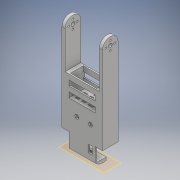
# Autodesk Inventor part: arm_1
Saved by Autodesk Inventor 2018 (Build 220112000, 112)
## iProperties
Created: 2018-02-05
Part Number: arm_1
Material: Genérico
Document SubType Name: Modeling
Designer: se_ma
Density: 1 g/cm^3
Appearance: Valor por defecto
Author: se_ma
Autodesk Inventor part; units mm, degrees
ref_plane "YZ Plane" through (0, 0, 0) normal (1, 0, 0) x (0, 1, 0)
ref_plane "XZ Plane" through (0, 0, 0) normal (0, 1, 0) x (-1, 0, 0)
ref_plane "XY Plane" through (0, 0, 0) normal (0, 0, 1) x (1, 0, 0)
sketch "Boceto1" plane through (0, 0, 0) normal (0, 1, 0) x (-1, 0, 0)
  line L0 (0, 0) -> (60, 0)
  line L1 (60, 0) -> (60, -80)
  line L2 (60, -80) -> (0, -80)
  line L3 (0, -80) -> (0, 0)
  dimension "d0" = 60
  dimension "d1" = 80
  constraints: 8 end point, 2 parallel, 1 horizontal, 1 perpendicular
  measures "d0" distance of L1.end L2.end
  measures "d1" distance of L0.end L1.end
extrude "Extrusión1" add sketch "Boceto1" along normal blind 25
sketch "Boceto2" plane through (-60, 0, 0) normal (0, 0, 1) x (1, 0, 0)
  line L0 (0, 25) -> (60, 25) projected
  line L1 (30, 25) -> (30, 23)
  line L2 (60, 0) -> (0, 0) projected
  line L3 (30, 0) -> (30, 2)
  line L4 (0, 0) -> (0, 25) projected
  line L5 (60, 0) -> (60, 25) projected
  line L6 (30, 23) -> (9, 23)
  line L7 (9, 2) -> (30, 2)
  line L8 (30, 23) -> (51, 23)
  line L9 (51, 2) -> (30, 2)
  line L10 (9, 23) -> (9, 19.5)
  line L11 (9, 2) -> (9, 5.5)
  arc A0 (9, 19.5) -> (1, 12.5) centre (7.9996, 12.5719) ccw
  arc A1 (1, 12.5) -> (9, 5.5) centre (7.9996, 12.4281) ccw
  line L12 (51, 23) -> (51, 19.5)
  line L13 (51, 2) -> (51, 5.5)
  arc A2 (59, 12.5) -> (51, 19.5) centre (52.0004, 12.5719) ccw
  arc A3 (51, 5.5) -> (59, 12.5) centre (52.0004, 12.4281) ccw
  dimension "d4" = 2
  dimension "d5" = 2
  dimension "d7" = 21
  dimension "d12" = 3.5
  dimension "d13" = 3.5
  dimension "d15" = 7
  dimension "d16" = 7
  dimension "d17" = 3.5
  dimension "d18" = 3.5
  dimension "d19" = 7
  dimension "d20" = 7
  constraints: 20 end point, 8 point on circle, 5 vertical, 4 centre point, 2 midpoint, 2 point on line, 1 horizontal
  measures "d4" distance of L1.start L1.end
  measures "d5" distance of L3.start L3.end
  measures "d7" distance of L1.end L8.end
  measures "d12" distance of L6.end L10.end
  measures "d13" distance of L7.start L11.end
  measures "d15" radius of A0
  measures "d16" radius of A1
  measures "d17" distance of L8.end L12.end
  measures "d18" distance of L9.start L13.end
  measures "d19" radius of A2
  measures "d20" radius of A3
extrude "Extrusión2" cut sketch "Boceto2" against normal blind 80 contours L8 L12 A2 A3 L13 L9 L7 L11 A1 A0 L10 L6
move faces "Desplazar1" translate (-1, 0, 0) faces at (-60, 8.3333, -26.6667)
move faces "Desplazar2" translate (1, 0, 0) faces at (0, 8.3333, -53.3333)
sketch "Boceto3" plane through (1, 0, 0) normal (1, 0, 0) x (0, 0, -1)
  line L0 (0, 0) -> (80, 0) projected
  line L1 (80, 0) -> (80, 25) projected
  line L2 (80, 0) -> (80, 25)
  line L3 (80, 25) -> (-60, 25)
  circle A0 centre (-60, 19.5) radius 1.5
  circle A1 centre (-67, 12.5) radius 1.5
  circle A2 centre (-60, 5.5) radius 1.5
  circle A3 centre (-53, 12.5) radius 1.5
  circle A4 centre (-60, 12.5) radius 3
  line L4 (80, 0) -> (-60, 0)
  arc A5 (-60, 25) -> (-60, 0) centre (-60, 12.5) ccw
  dimension "d29" = 25
  dimension "d30" = 140
  dimension "d35" = 3
  dimension "d36" = 3
  dimension "d37" = 3
  dimension "d38" = 3
  dimension "d39" = 6
  constraints: 6 centre point, 6 end point, 2 point on circle, 1 coincident, 1 horizontal, 1 perpendicular, 1 vertical
  measures "d29" distance of L0.end L1.end
  measures "d30" distance of L1.end L3.end
  measures "d35" diameter of A0
  measures "d36" diameter of A1
  measures "d37" diameter of A2
  measures "d38" diameter of A3
  measures "d39" diameter of A4
extrude "Extrusión3" add sketch "Boceto3" along normal blind 5
sketch "Boceto5" plane through (-61, 0, -80) normal (-1, 0, 0) x (0, 0, 1)
  line L0 (0, 0) -> (0, 25) projected
  line L1 (0, 0) -> (0, 25)
  line L2 (0, 25) -> (140, 25)
  line L3 (0, 0) -> (140, 0)
  circle A0 centre (140, 12.5) radius 3 projected
  circle A1 centre (140, 12.5) radius 3
  circle A2 centre (140, 19.5) radius 1.5
  circle A3 centre (133, 12.5) radius 1.5
  circle A4 centre (147, 12.5) radius 1.5
  circle A5 centre (140, 5.5) radius 1.5
  arc A6 (140, 0) -> (140, 25) centre (140, 12.5) ccw
  point P0 (80, 0)
  dimension "d52" = 3
  dimension "d53" = 3
  dimension "d54" = 3
  dimension "d55" = 3
  constraints: 6 centre point, 6 end point, 2 coincident, 2 point on circle, 1 horizontal, 1 perpendicular, 1 vertical
  measures "d52" diameter of A2
  measures "d53" diameter of A3
  measures "d54" diameter of A4
  measures "d55" diameter of A5
extrude "Extrusión4" add sketch "Boceto5" along normal blind 5
sketch "Boceto7" plane through (6, 0, -80) normal (0, 0, -1) x (-1, 0, 0)
  line L0 (57, 2) -> (15, 2) projected
  line L1 (57, 2) -> (65, 2)
  line L2 (65, 2) -> (65, 23)
  line L3 (57, 23) -> (15, 23) projected
  line L4 (65, 23) -> (57, 23)
  line L5 (57, 23) -> (57, 2)
  line L6 (15, 2) -> (7, 2)
  line L7 (7, 2) -> (7, 23)
  line L8 (7, 23) -> (15, 23)
  line L9 (15, 2) -> (15, 5.5) projected
  line L10 (15, 2) -> (15, 23)
  point P0 (6, 0)
  dimension "d60" = 8
  dimension "d61" = 21
  dimension "d62" = 8
  constraints: 16 end point, 5 perpendicular, 2 horizontal
  measures "d60" distance of L0.start L1.end
  measures "d61" distance of L1.end L2.end
  measures "d62" distance of L0.end L6.end
extrude "Extrusión5" add sketch "Boceto7" against normal blind 80 contours L5 L4 L2 L1 | L6 L7 L8 L10 L9
move faces "Desplazar3" translate (3.5, 0, 0) faces at (-61, 12.5, 17.1667) (-66, 12.5, -36.1667)
move faces "Desplazar4" translate (-3.5, 0, 0) faces at (1, 12.5, 17.1667) (6, 12.5, -36.1667)
sketch "Boceto11" plane through (0, 25, 0) normal (0, 1, 0) x (1, 0, 0)
  line L0 (-62.5, 80) -> (2.5, 80) projected
  line L1 (-51, 0) -> (-51, 80) projected
  line L2 (-62.5, 80) -> (-51, 80)
  line L3 (-51, 80) -> (-51, 63)
  line L4 (-51, 0) -> (-51, 80) projected
  line L5 (-51, 63) -> (-9, 63)
  line L6 (-9, 0) -> (-9, 80) projected
  point P0 (0, 0)
  dimension "d104" = 17
  constraints: 6 end point, 2 perpendicular, 2 point on line
  measures "d104" distance of L1.end L3.end
extrude "Extrusión9" cut sketch "Boceto11" against normal blind 23
sketch "Boceto12" plane through (0, 25, 0) normal (0, 1, 0) x (1, 0, 0)
  line L0 (-51, 0) -> (-51, 63) projected
  line L1 (-51, 63) -> (-51, 0)
  line L2 (-9, 0) -> (-9, 63) projected
  line L3 (-51, 63) -> (-9, 63)
  line L4 (-9, 63) -> (-9, 0)
  line L5 (-9, 0) -> (-51, 0)
  point P0 (0, 0)
  constraints: 8 end point, 2 collinear, 1 horizontal, 1 perpendicular
extrude "Extrusión10" add sketch "Boceto12" against normal blind 23
sketch "Boceto13" plane through (0, 0, 0) normal (0, -1, 0) x (1, 0, 0)
  line L0 (-62.5, -80) -> (2.5, -80) projected
  line L1 (-51, -63) -> (-51, -80) projected
  line L2 (-62.5, -80) -> (-51, -80)
  line L3 (-51, -80) -> (-51, -103)
  line L4 (-51, -103) -> (-9, -103)
  line L5 (-9, -63) -> (-9, -80) projected
  line L6 (-9, -103) -> (-9, -80)
  line L7 (-9, -80) -> (-51, -80)
  point P0 (0, 0)
  dimension "d109" = 23
  dimension "d110" = 42
  constraints: 10 end point, 1 horizontal, 1 perpendicular, 1 vertical
  measures "d109" distance of L1.end L3.end
  measures "d110" distance of L3.end L4.end
extrude "Extrusión11" add sketch "Boceto13" against normal blind 2
sketch "Boceto14" plane through (-51, 0, -103) normal (-1, 0, 0) x (0, 0, 1)
  line L0 (23, 25) -> (163, 25) projected
  arc A0 (0, 25) -> (0, 0) centre (11.5217, 12.5) ccw
  line L1 (0, 0) -> (0, 2) projected
  line L2 (0, 0) -> (0, 12.5)
  line L3 (0, 12.5) -> (0, 17.5)
  line L4 (0, 17.5) -> (-4.7264, 17.5)
  point P0 (103, 0)
  dimension "d114" = 17
  dimension "d115" = 5
  constraints: 6 end point, 3 point on circle, 1 centre point, 1 perpendicular, 1 vertical
  measures "d114" radius of A0
  measures "d115" distance of L2.end L3.end
extrude "Extrusión12" add sketch "Boceto14" against normal blind 42
ref_plane "Plano de trabajo1" through (-51, 12.5, -108.4783) normal (0, 0, 1) x (1, 0, 0)
sketch "Boceto15" plane through (-51, 12.5, -108.4783) normal (0, 0, 1) x (1, 0, 0)
  line L0 (0, 5) -> (42, 5) projected
  line L1 (42, 5) -> (0, 5)
  line L2 (0, 5) -> (15, 5)
  line L3 (15, 5) -> (15, -7)
  line L4 (42, 5) -> (42, -10.5) projected
  line L5 (42, 5) -> (27, 5)
  line L6 (27, 5) -> (27, -7)
  line L7 (27, -7) -> (15, -7)
  point P0 (51, -12.5)
  dimension "d120" = 15
  dimension "d121" = 12
  dimension "d122" = 15
  constraints: 12 end point, 3 perpendicular, 2 point on line, 1 collinear
  measures "d120" distance of L0.start L2.end
  measures "d121" distance of L2.end L3.end
  measures "d122" distance of L0.end L5.end
extrude "Extrusión13" cut sketch "Boceto15" along normal blind 2.5
sketch "Boceto16" plane through (-51, 2, -103) normal (0, 0, 1) x (1, 0, 0)
  line L0 (0, 15.5) -> (42, 15.5) projected
  line L1 (0, 15.5) -> (42, 15.5)
  line L2 (21, 15.5) -> (21, 9.5)
  circle A0 centre (21, 9.5) radius 1.5
  point P0 (51, -2)
  dimension "d125" = 6
  dimension "d126" = 3
  constraints: 4 end point, 1 centre point, 1 coincident, 1 horizontal, 1 midpoint, 1 vertical
  measures "d125" distance of L2.start L2.end
  measures "d126" diameter of A0
extrude "Extrusión14" cut sketch "Boceto16" against normal blind 3
sketch "Boceto17" plane through (-51, 2, -103) normal (0, 0, 1) x (1, 0, 0)
  circle A0 centre (21, 9.5) radius 1.5 projected
  line L0 (21, 9.5) -> (18, 9.5)
  line L1 (18, 9.5) -> (17.6, 9.5)
  line L2 (17.6, 9.5) -> (19.3, 12.4445)
  line L3 (19.3, 12.4445) -> (22.7, 12.4445)
  line L4 (22.7, 12.4445) -> (24.4, 9.5)
  line L5 (24.4, 9.5) -> (22.7, 6.5555)
  line L6 (22.7, 6.5555) -> (19.3, 6.5555)
  line L7 (19.3, 6.5555) -> (17.6, 9.5)
  point P0 (51, -2)
  dimension "d129" = 3
  dimension "d131" = 0.4
  constraints: 16 end point, 2 horizontal, 1 coincident, 13 other
  measures "d129" distance of L0.start L0.end
  measures "d131" distance of L0.end L1.end
extrude "Extrusión15" cut sketch "Boceto17" against normal blind 1.9
sketch "Boceto18" plane through (0, 25, 0) normal (0, 1, 0) x (1, 0, 0)
  line L0 (-51, 63) -> (-51, 80) projected
  line L1 (-51, 63) -> (-51, 53)
  line L2 (-51, 53) -> (-57, 53)
  line L3 (-57, 53) -> (-57, 43)
  line L4 (-9, 43) -> (-3, 43)
  line L5 (-3, 43) -> (-3, 53)
  line L6 (-3, 53) -> (-9, 53)
  line L7 (-9, 63) -> (-9, 80) projected
  line L8 (-9, 53) -> (-9, 63)
  line L9 (-51, 63) -> (-9, 63) projected
  line L10 (-51, 63) -> (-9, 63)
  line L11 (-30, 33) -> (-35, 33)
  line L12 (-35, 33) -> (-35, 43)
  line L13 (-30, 33) -> (-25, 33)
  line L14 (-25, 33) -> (-25, 43)
  line L15 (-57, 43) -> (-35, 43)
  line L16 (-25, 43) -> (-9, 43)
  point P0 (0, 0)
  dimension "d134" = 10
  dimension "d135" = 6
  dimension "d136" = 10
  dimension "d137" = 6
  dimension "d138" = 10
  dimension "d141" = 5
  dimension "d142" = 5
  constraints: 28 end point, 3 horizontal, 3 perpendicular, 2 point on line, 1 collinear, 1 vertical
  measures "d134" distance of L0.start L1.end
  measures "d135" distance of L1.end L2.end
  measures "d136" distance of L2.end L3.end
  measures "d137" distance of L4.start L4.end
  measures "d138" distance of L4.end L5.end
  measures "d141" distance of L11.start L11.end
  measures "d142" distance of L11.start L13.end
extrude "Extrusión16" cut sketch "Boceto18" against normal blind 2
sketch "Boceto19" plane through (0, 25, 0) normal (0, 1, 0) x (1, 0, 0)
  line L0 (-35, 43) -> (-57, 43) projected
  line L1 (-51.0758, 43) -> (-51.0758, 0)
  line L2 (-57.5, 0) -> (-2.5, 0) projected
  line L3 (-3, 43) -> (-25, 43) projected
  line L4 (-8.8093, 43) -> (-8.8093, 0)
  line L5 (-25, 33) -> (-35, 33) projected
  line L6 (-35, 33) -> (-51.0758, 33)
  line L7 (-25, 33) -> (-8.8093, 33)
  line L8 (-51.0758, 33) -> (-51.0758, 24.75)
  line L9 (-51.0758, 24.75) -> (-51.0758, 16.5)
  line L10 (-51.0758, 16.5) -> (-51.0758, 8.25)
  line L11 (-51.0758, 8.25) -> (-8.8093, 8.25)
  line L12 (-51.0758, 16.5) -> (-8.8093, 16.5)
  line L13 (-51.0758, 24.75) -> (-8.8093, 24.75)
  point P0 (0, 0)
  dimension "d145" = 8.25
  dimension "d146" = 8.25
  dimension "d147" = 8.25
  constraints: 20 end point, 12 point on line, 5 perpendicular, 1 vertical
  measures "d145" distance of L6.end L8.end
  measures "d146" distance of L8.end L9.end
  measures "d147" distance of L9.end L10.end
extrude "Extrusión17" cut sketch "Boceto19" against normal blind 25 contours L6 L5 L7 L4 L13 L1 | L12 L4 L11 L1
sketch "Boceto20" plane through (-57.5, 0, 0) normal (0, 0, 1) x (1, 0, 0)
  line L0 (0, 25) -> (6.4242, 25)
  line L1 (6.4242, 23) -> (6.4242, 2)
  line L2 (6.4242, 25) -> (6.4242, 0) projected
  line L3 (6.4242, 23) -> (48.6907, 23)
  line L4 (48.6907, 25) -> (48.6907, 0) projected
  line L5 (48.6907, 23) -> (48.6907, 2)
  line L6 (48.6907, 2) -> (6.4242, 2)
  point P0 (57.5, 0)
  dimension "d150" = 2
  dimension "d151" = 21
  constraints: 10 end point, 2 horizontal, 2 point on line, 1 perpendicular, 1 vertical
  measures "d150" distance of L0.end L1.start
  measures "d151" distance of L1.start L1.end
extrude "Extrusión18" cut sketch "Boceto20" against normal blind 33
sketch "Boceto21" plane through (-25, 25, -33) normal (0, 0, 1) x (1, 0, 0)
  line L0 (16.1907, -25) -> (-26.0758, -25) projected
  line L1 (-26.0758, -25) -> (-26.0758, -20)
  line L2 (-26.0758, 0) -> (-26.0758, -25) projected
  line L3 (-26.0758, -20) -> (-21.0758, -20)
  line L4 (-21.0758, -20) -> (-21.0758, -5)
  line L5 (-21.0758, -20) -> (-16.0758, -20)
  line L6 (-16.0758, -20) -> (-16.0758, -5)
  line L7 (16, -2) -> (16, -23) projected
  line L8 (16, -5) -> (6, -5)
  line L9 (16, -5) -> (26, -5) construction
  line L10 (6, -5) -> (6, -20)
  line L11 (6, -20) -> (-16.0758, -20)
  line L12 (-16.0758, -5) -> (6, -5)
  line L13 (-21.0758, -5) -> (-16.0758, -5)
  line L14 (6, -5) -> (11, -5)
  line L15 (11, -5) -> (11, -20)
  line L16 (11, -20) -> (6, -20)
  line L17 (-16.0758, -20) -> (-11.0758, -20)
  line L18 (-11.0758, -20) -> (-11.0758, -5)
  line L19 (-11.0758, -20) -> (-6.0758, -20)
  line L20 (-6.0758, -20) -> (-6.0758, -5)
  line L21 (-6.0758, -20) -> (-1.0758, -20)
  line L22 (-1.0758, -20) -> (-1.0758, -5)
  point P0 (25, -25)
  dimension "d154" = 5
  dimension "d155" = 5
  dimension "d156" = 15
  dimension "d157" = 5
  dimension "d158" = 10
  dimension "d159" = 180
  dimension "d160" = 15
  dimension "d161" = 5
  dimension "d162" = 5
  dimension "d163" = 5
  dimension "d164" = 5
  constraints: 40 end point, 11 perpendicular, 8 point on line, 2 collinear, 2 horizontal, 1 midpoint
  measures "d154" distance of L0.end L1.end
  measures "d155" distance of L1.end L3.end
  measures "d156" distance of L3.end L4.end
  measures "d157" distance of L3.end L5.end
  measures "d158" distance of L8.start L8.end
  measures "d159" angle of L8 L9
  measures "d160" distance of L8.end L10.end
  measures "d161" distance of L8.end L14.end
  measures "d162" distance of L5.end L17.end
  measures "d163" distance of L17.end L19.end
  measures "d164" distance of L19.end L21.end
extrude "Extrusión19" cut sketch "Boceto21" against normal blind 30 contours L4 L13 L6 L5 | L18 L12 L20 L11 | L22 L12 L10 L11
sketch "Boceto22" plane through (-51, 2, -63) normal (0, 1, 0) x (1, 0, 0)
  line L0 (42, 17) -> (42, 40) projected
  line L1 (42, 40) -> (38, 40)
  line L2 (42, 40) -> (0, 40) projected
  line L3 (38, 40) -> (38, 31)
  line L4 (38, 31) -> (31, 31)
  line L5 (31, 31) -> (31, 19)
  line L6 (31, 19) -> (38, 19)
  line L7 (38, 19) -> (38, 31)
  point P0 (51, -63)
  dimension "d167" = 4
  dimension "d168" = 9
  dimension "d169" = 7
  dimension "d170" = 12
  constraints: 12 end point, 5 perpendicular, 2 point on line
  measures "d167" distance of L0.end L1.end
  measures "d168" distance of L1.end L3.end
  measures "d169" distance of L3.end L4.end
  measures "d170" distance of L4.end L5.end
extrude "Extrusión20" cut sketch "Boceto22" against normal blind 2
sketch "Boceto23" plane through (0, 23, 0) normal (0, 1, 0) x (1, 0, 0)
  line L0 (-51, 63) -> (-51, 80) projected
  line L1 (-51, 63) -> (-51, 43)
  line L2 (-35, 43) -> (-57, 43) projected
  line L3 (-51, 53) -> (-51, 80) projected
  line L4 (-9, 80) -> (-9, 53) projected
  line L5 (-30, 53) -> (-30, 63)
  line L6 (-41.0758, 33) -> (-41.0758, 63) projected
  line L7 (-19, 33) -> (-19, 63) projected
  line L8 (-36.0758, 33) -> (-36.0758, 63) projected
  line L9 (-36.0758, 53) -> (-41.0758, 53)
  circle A0 centre (-38.5758, 53) radius 1.5
  line L10 (-36.0758, 53) -> (-19, 53)
  line L11 (-19, 33) -> (-19, 63) projected
  line L12 (-19, 53) -> (-14, 53)
  circle A1 centre (-16.5, 53) radius 1.5
  point P0 (0, 0)
  dimension "d175" = 5
  dimension "d176" = 3
  dimension "d177" = 5
  dimension "d178" = 3
  constraints: 10 end point, 4 point on line, 2 centre point, 2 midpoint, 2 vertical, 1 perpendicular
  measures "d175" distance of L9.start L9.end
  measures "d176" diameter of A0
  measures "d177" distance of L10.end L12.end
  measures "d178" diameter of A1
extrude "Extrusión21" cut sketch "Boceto23" against normal blind 23 contours A0 L9 | L9 A0 | A1 L12 | L12 A1
sketch "Boceto24" plane through (0, 0, 0) normal (0, -1, 0) x (1, 0, 0)
  circle A0 centre (-38.5758, -53) radius 1.5 projected
  line L0 (-38.5758, -53) -> (-41.9758, -53)
  circle A1 centre (-16.5, -53) radius 1.5 projected
  line L1 (-16.5, -53) -> (-19.9, -53)
  line L2 (-41.9758, -53) -> (-40.2758, -50.0555)
  line L3 (-40.2758, -50.0555) -> (-36.8758, -50.0555)
  line L4 (-36.8758, -50.0555) -> (-35.1758, -53)
  line L5 (-35.1758, -53) -> (-36.8758, -55.9445)
  line L6 (-36.8758, -55.9445) -> (-40.2758, -55.9445)
  line L7 (-40.2758, -55.9445) -> (-41.9758, -53)
  line L8 (-19.9, -53) -> (-18.2, -50.0555)
  line L9 (-18.2, -50.0555) -> (-14.8, -50.0555)
  line L10 (-14.8, -50.0555) -> (-13.1, -53)
  line L11 (-13.1, -53) -> (-14.8, -55.9445)
  line L12 (-14.8, -55.9445) -> (-18.2, -55.9445)
  line L13 (-18.2, -55.9445) -> (-19.9, -53)
  point P0 (0, 0)
  dimension "d181" = 3.4
  dimension "d182" = 3.4
  constraints: 28 end point, 2 coincident, 2 horizontal, 26 other
  measures "d181" distance of L0.start L0.end
  measures "d182" distance of L1.start L1.end
extrude "Extrusión22" cut sketch "Boceto24" against normal blind 1.9
